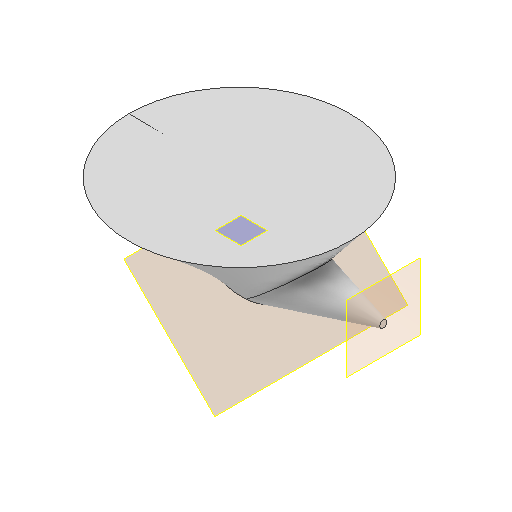
# Autodesk Inventor part: 00_beam
Saved by Autodesk Inventor 2022.5 (Build 265521000, 521)
## iProperties
Created: 2023-11-03
Part Number: 00_beam
Material: Generisch
Document SubType Name: Modeling
Designer: diederichbenedict
Density: 1 g/cm^3
Appearance: Vorgabe
Author: diederichbenedict
Autodesk Inventor part; units mm, degrees
ref_plane "Arbeitsebene7" through (-216.5727, -10, -25) normal (1, 0, 0) x (0, 0, 1)
sketch "Skizze5" plane through (-216.5727, -10, -25) normal (1, 0, 0) x (0, 0, 1)
  line L0 (7.88, 8) -> (7.88, 42.1) projected
  line L1 (47.8, 8) -> (7.88, 8) projected
  line L2 (41.92, 42.1) -> (41.92, 8) projected
  line L3 (2, 42.1) -> (41.92, 42.1) projected
  circle A0 centre (24.9, 25.02) radius 17.02
  circle A1 centre (24.9, 25.02) radius 2.5
  point P0 (25, -10)
  dimension "d12" = 5
  constraints: 3 tangent, 2 centre point, 1 coincident
  measures "d12" diameter of A1
ref_plane "Arbeitsebene8" through (-325.7058, -30.7243, -60) normal (0.7071068, 0.7071068, 0) x (0, 0, 1)
ref_plane "Arbeitsebene10" through (-297.9374, -51.4217, -57.555) normal (0.7071068, 0.7071068, 0) x (-0.7071068, 0.7071068, 0)
ref_plane "Arbeitsebene12" through (-294.4018, -47.8861, -57.555) normal (0.7071068, 0.7071068, 0) x (-0.7071068, 0.7071068, 0)
extrude "Extrusion5" add sketch "Skizze5" against normal up to surface draft 15 contours A1 surface through (-294.4018, -47.8861, -57.555) normal (0.7071068, 0.7071068, 0)
ref_plane "Arbeitsebene9" through (-282.9372, 2.56, 30.775) normal (0, -1, 0) x (0, 0, 1)
sketch "Skizze6" plane through (-282.9372, 2.56, 30.775) normal (0, -1, 0) x (0, 0, 1)
  ellipse E0 centre (-30.875, 32.0678) end of major axis (-30.875, 60.9426) minor radius 27.819 projected
  arc A0 (-91.72, 71.76) -> (-94.72, 68.76) centre (-91.72, 68.76) ccw projected
  arc A1 (-94.72, -10.84) -> (-91.72, -13.84) centre (-91.72, -10.84) ccw projected
  arc A2 (28.67, -12.34) -> (31.67, -9.34) centre (28.67, -9.34) ccw projected
  arc A3 (31.67, 67.26) -> (28.67, 70.26) centre (28.67, 67.26) ccw projected
  circle A4 centre (-30.875, 32.0678) radius 75.5265
  point P0 (-30.775, -282.9372)
  constraints: 1 centre point, 1 coincident
ref_plane "Arbeitsebene11" through (-294.4018, -47.8861, 2.445) normal (0.7071068, 0.7071068, 0) x (0.7071068, -0.7071068, 0)
sketch "Skizze7" plane through (-294.4018, -47.8861, 2.445) normal (0.7071068, 0.7071068, 0) x (0.7071068, -0.7071068, 0)
  ellipse E0 centre (-29.1372, 2.545) end of major axis (-69.9724, 2.545) minor radius 27.819 projected
  point P0 (174.3129, 2.445)
  constraints: 1 other
loft "Erhebung1" add profiles "Skizze6", "Skizze7" contours E0 | A4 / all
